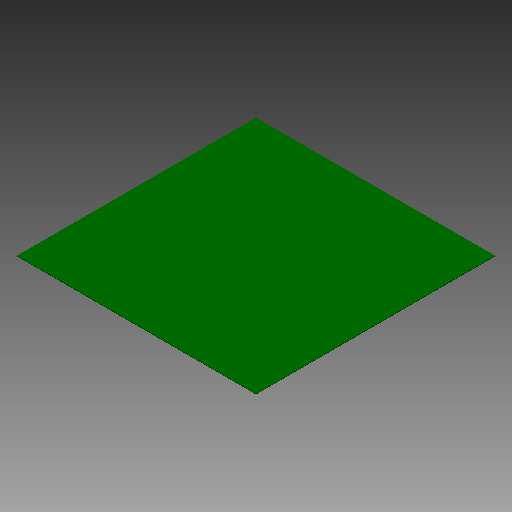
# Autodesk Inventor part: Ground
Saved by Autodesk Inventor 2018 (Build 220112000, 112)
## iProperties
Created: 2016-01-10
Part Number: Ground
Material: Generic
Document SubType Name: Modeling
Designer: Applefamily
Density: 1 g/cm^3
Appearance: Default
Author: Applefamily
Autodesk Inventor part; units mm, degrees
ref_plane "YZ Plane" through (0, 0, 0) normal (1, 0, 0) x (0, 1, 0)
ref_plane "XZ Plane" through (0, 0, 0) normal (0, 1, 0) x (-1, 0, 0)
ref_plane "XY Plane" through (0, 0, 0) normal (0, 0, 1) x (1, 0, 0)
sketch "Sketch1" plane through (0, 0, 0) normal (0, 1, 0) x (-1, 0, 0)
  line L0 (-26.023, -13.7591) -> (989.977, -13.7591)
  line L1 (989.977, -13.7591) -> (989.977, 1002.2409)
  line L2 (989.977, 1002.2409) -> (-26.023, 1002.2409)
  line L3 (-26.023, 1002.2409) -> (-26.023, -13.7591)
  point P0 (0, 0)
  dimension "d0" = 1016
  dimension "d1" = 1016
  constraints: 8 end point, 2 parallel, 1 horizontal, 1 perpendicular
  measures "d0" distance of L2.end L1.end
  measures "d1" distance of L1.end L0.end
extrude "Extrusion1" add sketch "Sketch1" along normal blind 2.54
body "Solid1"
